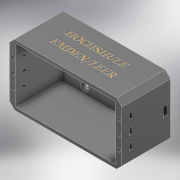
# Autodesk Inventor part: 3
Saved by Autodesk Inventor 2022 (Build 260153000, 153)
## iProperties
Company: HS Emden/Leer
Created: 2023-12-23
Part Number: 3
Material: PMMA-Kunststoff
Document SubType Name: Sheet Metal
Designer: Yaman Alsaady
Density: 1.188 g/cm^3
Appearance: Glatt - Schwarz
Sheet Metal Rule: Standard
Project: Delta-Robot
Author: Yaman Alsaady
Title: Case
## iProperties of the stored document 1_3D-Druck.ipt
Created: 2023-12-25
Part Number: 1_3D-Druck
Material: Generisch
Document SubType Name: Modeling
Designer: alsaa
Density: 1 g/cm^3
Appearance: Vorgabe
Author: alsaa
Autodesk Inventor part; units mm, degrees
(part 1 of 2)
ref_plane "YZ Plane" through (0, 0, 0) normal (1, 0, 0) x (0, 1, 0)
ref_plane "XZ Plane" through (0, 0, 0) normal (0, 1, 0) x (-1, 0, 0)
ref_plane "XY Plane" through (0, 0, 0) normal (0, 0, 1) x (1, 0, 0)
sketch "Skizze1" plane through (0, 0, 0) normal (0, 0, 1) x (1, 0, 0)
  line L0 (-30.75, -10.25) -> (10.25, -10.25)
  line L1 (10.25, -10.25) -> (10.25, 10.25)
  line L2 (10.25, 10.25) -> (-30.75, 10.25)
  line L3 (-30.75, 10.25) -> (-30.75, -10.25)
  line L4 (0, -10.25) -> (0, 10.25)
  circle A0 centre (-34.5, -5) radius 2.15
  circle A1 centre (-34.5, 5) radius 2.15
  circle A2 centre (14, 5) radius 2.15
  circle A3 centre (14, -5) radius 2.15
  line L5 (-10.25, -10.25) -> (-10.25, 10.25)
  line L6 (-56, 0) -> (56, 0)
  line L7 (53, 29) -> (-53, 29)
  line L8 (-53, 29) -> (-53, -29)
  line L9 (-53, -29) -> (53, -29)
  line L10 (53, -29) -> (53, 29)
  line L11 (53, 29) -> (-53, -29) construction
  line L12 (-53, 29) -> (53, -29) construction
  line L13 (-53, -10.25) -> (53, -10.25)
  line L14 (-53, 10.25) -> (53, 10.25)
  point P0 (0, 0)
  point P1 (0, 0)
  point P2 (0, 0)
  dimension "d8" = 48.5
  dimension "d9" = 4.3
  dimension "d10" = 20.5
  dimension "d11" = 41
  dimension "d12" = 34.5
  dimension "d13" = 10
  dimension "d14" = 58
  dimension "d15" = 106
  dimension "d18" = 20.5
  constraints: 30 end point, 6 midpoint, 6 parallel, 4 centre point, 4 horizontal, 4 point on line, 4 symmetric about line, 3 equal radius, 3 perpendicular, 2 coincident, 1 other
  measures "d8" distance of A2.centre A1.centre
  measures "d9" diameter of A0
  measures "d10" distance of L1.start L1.end
  measures "d11" distance of L0.start L1.start
  measures "d12" horizontal distance of L4.start A0.centre
  measures "d13" distance of A2.centre A3.centre
  measures "d14" distance of L9.end L7.start
  measures "d15" distance of L8.end L9.end
  measures "d18" distance between parallel lines of L14 L13
extrude "Extrusion1" add sketch "Skizze1" along normal blind 3 contours L3 L6 L5 L0 | L13 L8 L6 L3 | L0 L13 L10 L9 L8 | L5 L6 L4 L0 | L6 L8 L14 L3 | L3 L2 L5 L6 | L4 L6 L1 L0 | L5 L2 L4 L6 | L14 L8 L7 L10 L2 | L1 L6 L10 L13 | L4 L2 L1 L6 | L1 L14 L10 L6 | A0 | A1 | A2 | A3
sketch "Skizze2" plane through (0, 0, 3) normal (0, 0, 1) x (1, 0, 0)
  line L0 (53, 29) -> (-53, 29) projected
  line L1 (-53, -29) -> (53, -29) projected
  line L2 (-53, 29) -> (-47, 29)
  line L3 (-47, 29) -> (-47, -29)
  line L4 (-47, -29) -> (-53, -29)
  line L5 (-53, -29) -> (-53, 29)
  line L6 (53, -29) -> (53, 29) projected
  line L7 (53, 29) -> (47, 29)
  line L8 (47, 29) -> (47, -29)
  line L9 (47, -29) -> (53, -29)
  line L10 (53, -29) -> (53, 29)
  point P0 (0, 0)
  dimension "d19" = 6
  dimension "d20" = 6
  constraints: 16 end point, 4 parallel, 2 horizontal, 2 perpendicular, 2 point on line
  measures "d19" distance between parallel lines of L3 L5
  measures "d20" distance between parallel lines of L6 L8
extrude "Extrusion2" add sketch "Skizze2" along normal blind 43 contours L6 L1 L8 L0 | L3 L1 L5 L0
sketch "Skizze3" plane through (0, 0, 46) normal (0, 0, 1) x (1, 0, 0)
  line L0 (-47, 29) -> (-53, 29) construction
  line L1 (-53, 29) -> (-47, 29) construction
  line L2 (-47, 29) -> (-50, 29) construction
  line L3 (-50, 29) -> (-50, -29) construction
  line L4 (-53, 29) -> (-53, -29) construction
  line L5 (53, 29) -> (-53, 29) construction
  line L6 (0, 29) -> (0, -30.13) construction
  line L7 (-53, 0) -> (-47, 0) construction
  line L8 (-47, 29) -> (-47, -29) construction
  circle A0 centre (-50, 12.5) radius 1.85
  circle A1 centre (-50, -12.5) radius 1.85
  circle A2 centre (50, 12.5) radius 1.85
  circle A3 centre (50, -12.5) radius 1.85
  circle A4 centre (-50, 0) radius 1.85
  circle A5 centre (50, 0) radius 1.85
  point P0 (0, 0)
  dimension "d24" = 25
  dimension "d33" = 3.7
  constraints: 10 end point, 6 centre point, 5 midpoint, 4 symmetric about line, 2 equal length, 2 equal radius, 2 point on line, 1 vertical, 3 other
  measures "d24" distance of A1.centre A0.centre
  measures "d33" diameter of A4
extrude "Extrusion3" cut sketch "Skizze3" against normal blind 20
sketch "Skizze4" plane through (0, 0, 3) normal (0, 0, 1) x (1, 0, 0)
  line L0 (25, -20) -> (-25, -20)
  line L1 (-25, -20) -> (-25, 20)
  line L2 (-25, 20) -> (25, 20)
  line L3 (25, 20) -> (25, -20)
  line L4 (25, -20) -> (-25, 20) construction
  line L5 (-25, -20) -> (25, 20) construction
  circle A0 centre (-25, 20) radius 1.85
  circle A1 centre (25, 20) radius 1.85
  circle A2 centre (25, -20) radius 1.85
  circle A3 centre (-25, -20) radius 1.85
  point P0 (0, 0)
  dimension "d27" = 50
  dimension "d28" = 40
  dimension "d29" = 3.7
  constraints: 12 end point, 4 centre point, 4 coincident, 3 equal radius, 2 midpoint, 2 parallel, 1 horizontal, 1 perpendicular
  measures "d27" distance of L1.end L2.end
  measures "d28" distance of L2.end L0.start
  measures "d29" diameter of A1
extrude "Extrusion4" cut sketch "Skizze4" against normal through all contours A3 L1 L0 | L0 L1 A3 | A2 L3 L0 | L0 L3 A2 | A0 L2 L1 | L1 L2 A0 | A1 L2 L3 | L3 L2 A1
fillet "Rundung1" radius 2 4 edges at (-26.85, 20, 3) (23.15, 20, 3) (23.15, -20, 3) (-26.85, -20, 3)
sketch "Skizze5" plane through (0, 0, 3) normal (0, 0, 1) x (1, 0, 0)
  line L0 (-47, -29) -> (-47, 29) projected
  line L1 (-47, 26) -> (47, 26)
  line L2 (47, -29) -> (47, 29) projected
  line L3 (-47, -26) -> (47, -26)
  line L4 (-47, -29) -> (47, -29) projected
  line L5 (47, 29) -> (-47, 29) projected
  point P0 (0, 0)
  dimension "d34" = 3
  dimension "d35" = 3
  constraints: 4 end point, 2 horizontal, 2 point on line
  measures "d34" distance between parallel lines of L4 L3
  measures "d35" distance between parallel lines of L1 L5
extrude "Extrusion5" add sketch "Skizze5" along normal up to surface (43 mm away) contours L0 L3 L2 L4 | L0 L5 L2 L1
chamfer "Fase1" distance 5 angle 45 4 edges at (53, 29, 23) (53, -29, 23) (-53, -29, 23) (-53, 29, 23)
sketch "Skizze6" plane through (-48, -29, 0) normal (0, -1, 0) x (1, 0, 0)
  line L0 (0, 0) -> (0, 46) projected
  line L1 (0, 0) -> (96, 0) projected
  line L2 (96, 46) -> (96, 0) projected
  line L3 (0, 46) -> (96, 46) projected
  line L4 (0, 0) -> (0, 46) construction
  line L5 (0, 23) -> (96, 23) construction
  line L6 (1, 46) -> (95, 46) construction
  line L7 (48, 46) -> (48, 0) construction
  line L8 (75.5, 12) -> (20.5, 12) construction
  line L9 (20.5, 12) -> (20.5, 34) construction
  line L10 (20.5, 34) -> (75.5, 34) construction
  line L11 (75.5, 34) -> (75.5, 12) construction
  line L12 (77.3044, 18.1442) -> (76.7258, 17.963)
  spline S0 degree 2 poles (76.7258, 17.963) (76.6351, 17.9351) (76.4957, 17.8026) (76.4678, 17.712) knots 0 0 0 1 2 2 2
  line L13 (76.4678, 17.712) -> (75.4361, 13.0481)
  spline S1 degree 2 poles (75.4361, 13.0481) (75.4151, 12.9505) (75.4988, 12.8181) (75.5825, 12.7972) knots 0 0 0 1 2 2 2
  line L14 (75.5825, 12.7972) -> (76.1681, 12.6159)
  line L15 (76.1681, 12.6159) -> (76.1053, 12.3301)
  line L16 (76.1053, 12.3301) -> (73.2819, 12.3301)
  line L17 (73.2819, 12.3301) -> (73.3446, 12.6159)
  line L18 (73.3446, 12.6159) -> (73.9163, 12.7972)
  spline S2 degree 2 poles (73.9163, 12.7972) (74.0069, 12.825) (74.1533, 12.9505) (74.1742, 13.0481) knots 0 0 0 1 2 2 2
  line L19 (74.1742, 13.0481) -> (74.6065, 14.9932)
  line L20 (74.6065, 14.9932) -> (72.0828, 14.9932)
  line L21 (72.0828, 14.9932) -> (71.6506, 13.0481)
  spline S3 degree 2 poles (71.6506, 13.0481) (71.6297, 12.9505) (71.7133, 12.8181) (71.797, 12.7972) knots 0 0 0 1 2 2 2
  line L22 (71.797, 12.7972) -> (72.3826, 12.6159)
  line L23 (72.3826, 12.6159) -> (72.3198, 12.3301)
  line L24 (72.3198, 12.3301) -> (69.4964, 12.3301)
  line L25 (69.4964, 12.3301) -> (69.5591, 12.6159)
  line L26 (69.5591, 12.6159) -> (70.1308, 12.7972)
  spline S4 degree 2 poles (70.1308, 12.7972) (70.2214, 12.825) (70.3609, 12.9575) (70.3887, 13.0481) knots 0 0 0 1 2 2 2
  line L27 (70.3887, 13.0481) -> (71.4205, 17.712)
  spline S5 degree 2 poles (71.4205, 17.712) (71.4414, 17.8096) (71.3578, 17.9421) (71.2741, 17.963) knots 0 0 0 1 2 2 2
  line L28 (71.2741, 17.963) -> (70.6885, 18.1442)
  line L29 (70.6885, 18.1442) -> (70.7513, 18.4301)
  line L30 (70.7513, 18.4301) -> (73.5817, 18.4301)
  line L31 (73.5817, 18.4301) -> (73.5119, 18.1442)
  line L32 (73.5119, 18.1442) -> (72.9403, 17.963)
  spline S6 degree 2 poles (72.9403, 17.963) (72.8497, 17.9351) (72.7033, 17.8026) (72.6823, 17.712) knots 0 0 0 1 2 2 2
  line L33 (72.6823, 17.712) -> (72.2013, 15.523)
  line L34 (72.2013, 15.523) -> (74.718, 15.523)
  line L35 (74.718, 15.523) -> (75.206, 17.712)
  spline S7 degree 2 poles (75.206, 17.712) (75.2269, 17.8096) (75.1363, 17.9421) (75.0526, 17.963) knots 0 0 0 1 2 2 2
  line L36 (75.0526, 17.963) -> (74.474, 18.1442)
  line L37 (74.474, 18.1442) -> (74.5437, 18.4301)
  line L38 (74.5437, 18.4301) -> (77.3602, 18.4301)
  line L39 (77.3602, 18.4301) -> (77.3044, 18.1442)
  spline S8 degree 2 poles (67.1819, 18.5695) (67.7884, 18.5695) (68.7156, 18.2279) (69.343, 17.6005) (69.6777, 16.7081) (69.6777, 16.1504) knots 0 0 0 1 2 3 4 4 4
  spline S9 degree 2 poles (69.6777, 16.1504) (69.6777, 15.6694) (69.4685, 14.7143) (69.0572, 13.8359) (68.4437, 13.076) (67.6559, 12.5183) (66.6869, 12.1976) (66.1222, 12.1976) knots 0 0 0 1 2 3 4 5 6 6 6
  spline S10 degree 2 poles (66.1222, 12.1976) (65.4948, 12.1976) (64.5606, 12.5532) (63.9402, 13.1945) (63.6195, 14.0729) (63.6195, 14.6028) knots 0 0 0 1 2 3 4 4 4
  spline S11 degree 2 poles (63.6195, 14.6028) (63.6195, 15.042) (63.8077, 15.9692) (64.1981, 16.8476) (64.7977, 17.6353) (65.5854, 18.2209) (66.5823, 18.5695) (67.1819, 18.5695) knots 0 0 0 1 2 3 4 5 6 6 6
  spline S12 degree 2 poles (67.0494, 18.0606) (66.7148, 18.0606) (66.1362, 17.7469) (65.6761, 17.2101) (65.3275, 16.499) (65.1044, 15.6973) (64.9859, 14.8468) (64.9859, 14.4494) knots 0 0 0 1 2 3 4 5 6 6 6
  spline S13 degree 2 poles (64.9859, 14.4494) (64.9859, 14.045) (65.1323, 13.3967) (65.439, 12.9436) (65.9131, 12.6996) (66.2477, 12.6996) knots 0 0 0 1 2 3 4 4 4
  spline S14 degree 2 poles (66.2477, 12.6996) (66.5893, 12.6996) (67.1679, 13.0272) (67.6281, 13.578) (67.9697, 14.296) (68.1927, 15.0838) (68.3043, 15.8855) (68.3043, 16.248) knots 0 0 0 1 2 3 4 5 6 6 6
  spline S15 degree 2 poles (68.3043, 16.248) (68.3043, 16.6454) (68.1718, 17.3077) (67.8721, 17.7887) (67.398, 18.0606) (67.0494, 18.0606) knots 0 0 0 1 2 3 4 4 4
  spline S16 degree 2 poles (60.7682, 18.5556) (61.3468, 18.5556) (62.267, 18.1861) (62.9014, 17.5029) (63.2361, 16.5408) (63.2361, 15.9552) knots 0 0 0 1 2 3 4 4 4
  spline S17 degree 2 poles (63.2361, 15.9552) (63.2361, 15.4463) (62.999, 14.4842) (62.5668, 13.6477) (61.9394, 12.9645) (61.1655, 12.4695) (60.2453, 12.2046) (59.7294, 12.2046) knots 0 0 0 1 2 3 4 5 6 6 6
  spline S18 degree 2 poles (59.7294, 12.2046) (59.5063, 12.2046) (58.9695, 12.2673) (58.4537, 12.3649) (58.0005, 12.4974) (57.8402, 12.5601) knots 0 0 0 1 2 3 4 4 4
  line L40 (57.8402, 12.5601) -> (58.126, 14.0799)
  line L41 (58.126, 14.0799) -> (58.4676, 14.0799)
  line L42 (58.4676, 14.0799) -> (58.6419, 13.2852)
  spline S19 degree 2 poles (58.6419, 13.2852) (58.6489, 13.2154) (58.7186, 13.1248) (58.7743, 13.0969) knots 0 0 0 1 2 2 2
  spline S20 degree 2 poles (58.7743, 13.0969) (58.8929, 13.0342) (59.1996, 12.9017) (59.5273, 12.8041) (59.8549, 12.7484) (59.9943, 12.7484) knots 0 0 0 1 2 3 4 4 4
  spline S21 degree 2 poles (59.9943, 12.7484) (60.3708, 12.7484) (61.047, 13.2294) (61.5629, 14.059) (61.8627, 15.1744) (61.8627, 15.8158) knots 0 0 0 1 2 3 4 4 4
  spline S22 degree 2 poles (61.8627, 15.8158) (61.8627, 16.2759) (61.6954, 17.0288) (61.3119, 17.5656) (60.7054, 17.8445) (60.2662, 17.8445) knots 0 0 0 1 2 3 4 4 4
  spline S23 degree 2 poles (60.2662, 17.8445) (60.0222, 17.8445) (59.5203, 17.6911) (59.0532, 17.475) (58.6419, 17.2101) (58.4815, 17.0985) knots 0 0 0 1 2 3 4 4 4
  line L43 (58.4815, 17.0985) -> (58.2724, 17.0985)
  line L44 (58.2724, 17.0985) -> (58.3909, 17.6144)
  spline S24 degree 2 poles (58.3909, 17.6144) (58.5931, 17.7748) (59.0881, 18.1024) (59.6737, 18.3813) (60.3638, 18.5556) (60.7682, 18.5556) knots 0 0 0 1 2 3 4 4 4
  line L45 (58.2933, 18.1442) -> (57.7147, 17.963)
  spline S25 degree 2 poles (57.7147, 17.963) (57.6241, 17.9351) (57.4846, 17.8026) (57.4567, 17.712) knots 0 0 0 1 2 2 2
  line L46 (57.4567, 17.712) -> (56.425, 13.0481)
  spline S26 degree 2 poles (56.425, 13.0481) (56.4041, 12.9505) (56.4877, 12.8181) (56.5714, 12.7972) knots 0 0 0 1 2 2 2
  line L47 (56.5714, 12.7972) -> (57.157, 12.6159)
  line L48 (57.157, 12.6159) -> (57.0942, 12.3301)
  line L49 (57.0942, 12.3301) -> (54.2708, 12.3301)
  line L50 (54.2708, 12.3301) -> (54.3335, 12.6159)
  line L51 (54.3335, 12.6159) -> (54.9052, 12.7972)
  spline S27 degree 2 poles (54.9052, 12.7972) (54.9958, 12.825) (55.1422, 12.9505) (55.1631, 13.0481) knots 0 0 0 1 2 2 2
  line L52 (55.1631, 13.0481) -> (55.5954, 14.9932)
  line L53 (55.5954, 14.9932) -> (53.0717, 14.9932)
  line L54 (53.0717, 14.9932) -> (52.6395, 13.0481)
  spline S28 degree 2 poles (52.6395, 13.0481) (52.6186, 12.9505) (52.7022, 12.8181) (52.7859, 12.7972) knots 0 0 0 1 2 2 2
  line L55 (52.7859, 12.7972) -> (53.3715, 12.6159)
  line L56 (53.3715, 12.6159) -> (53.3087, 12.3301)
  line L57 (53.3087, 12.3301) -> (50.4853, 12.3301)
  line L58 (50.4853, 12.3301) -> (50.5481, 12.6159)
  line L59 (50.5481, 12.6159) -> (51.1197, 12.7972)
  spline S29 degree 2 poles (51.1197, 12.7972) (51.2103, 12.825) (51.3498, 12.9575) (51.3777, 13.0481) knots 0 0 0 1 2 2 2
  line L60 (51.3777, 13.0481) -> (52.4094, 17.712)
  spline S30 degree 2 poles (52.4094, 17.712) (52.4303, 17.8096) (52.3467, 17.9421) (52.263, 17.963) knots 0 0 0 1 2 2 2
  line L61 (52.263, 17.963) -> (51.6774, 18.1442)
  line L62 (51.6774, 18.1442) -> (51.7402, 18.4301)
  line L63 (51.7402, 18.4301) -> (54.5706, 18.4301)
  line L64 (54.5706, 18.4301) -> (54.5009, 18.1442)
  line L65 (54.5009, 18.1442) -> (53.9292, 17.963)
  spline S31 degree 2 poles (53.9292, 17.963) (53.8386, 17.9351) (53.6922, 17.8026) (53.6713, 17.712) knots 0 0 0 1 2 2 2
  line L66 (53.6713, 17.712) -> (53.1902, 15.523)
  line L67 (53.1902, 15.523) -> (55.7069, 15.523)
  line L68 (55.7069, 15.523) -> (56.1949, 17.712)
  spline S32 degree 2 poles (56.1949, 17.712) (56.2158, 17.8096) (56.1252, 17.9421) (56.0415, 17.963) knots 0 0 0 1 2 2 2
  line L69 (56.0415, 17.963) -> (55.4629, 18.1442)
  line L70 (55.4629, 18.1442) -> (55.5326, 18.4301)
  line L71 (55.5326, 18.4301) -> (58.3491, 18.4301)
  line L72 (58.3491, 18.4301) -> (58.2933, 18.1442)
  spline S33 degree 2 poles (48.9028, 18.5695) (49.1607, 18.5695) (49.7045, 18.5068) (50.2622, 18.3952) (50.799, 18.2488) (51.0361, 18.1652) knots 0 0 0 1 2 3 4 4 4
  line L73 (51.0361, 18.1652) -> (50.7433, 16.4362)
  line L74 (50.7433, 16.4362) -> (50.3947, 16.4362)
  line L75 (50.3947, 16.4362) -> (50.2204, 17.3077)
  spline S34 degree 2 poles (50.2204, 17.3077) (50.2065, 17.3704) (50.1367, 17.482) (50.074, 17.5308) knots 0 0 0 1 2 2 2
  spline S35 degree 2 poles (50.074, 17.5308) (49.9415, 17.6353) (49.5233, 17.8166) (49.098, 17.9421) (48.7076, 18.0118) (48.5961, 18.0118) knots 0 0 0 1 2 3 4 4 4
  spline S36 degree 2 poles (48.5961, 18.0118) (48.359, 18.0118) (47.9129, 17.8724) (47.5573, 17.6005) (47.3412, 17.2101) (47.3412, 16.9452) knots 0 0 0 1 2 3 4 4 4
  spline S37 degree 2 poles (47.3412, 16.9452) (47.3412, 16.7639) (47.4667, 16.492) (47.6758, 16.2829) (47.9547, 16.1156) (48.1011, 16.0458) knots 0 0 0 1 2 3 4 4 4
  spline S38 degree 2 poles (48.1011, 16.0458) (48.3521, 15.9204) (48.8679, 15.6833) (49.1259, 15.5648) knots 0 0 0 1 2 2 2
  spline S39 degree 2 poles (49.1259, 15.5648) (49.3559, 15.4602) (49.7254, 15.1814) (49.9903, 14.8328) (50.1298, 14.3936) (50.1298, 14.1287) knots 0 0 0 1 2 3 4 4 4
  spline S40 degree 2 poles (50.1298, 14.1287) (50.1298, 13.808) (49.9206, 13.2712) (49.5581, 12.846) (49.0771, 12.5253) (48.5263, 12.3022) (47.9477, 12.1976) (47.6619, 12.1976) knots 0 0 0 1 2 3 4 5 6 6 6
  spline S41 degree 2 poles (47.6619, 12.1976) (47.4039, 12.1976) (46.902, 12.2464) (46.4001, 12.337) (45.9051, 12.4625) (45.6611, 12.5322) knots 0 0 0 1 2 3 4 4 4
  line L76 (45.6611, 12.5322) -> (45.9887, 14.1287)
  line L77 (45.9887, 14.1287) -> (46.3303, 14.1287)
  line L78 (46.3303, 14.1287) -> (46.4837, 13.313)
  spline S42 degree 2 poles (46.4837, 13.313) (46.5116, 13.2015) (46.6301, 13.1039) knots 0 0 0 1 1 1
  spline S43 degree 2 poles (46.6301, 13.1039) (46.7486, 13.0202) (47.0763, 12.8808) (47.4179, 12.7972) (47.7246, 12.7484) (47.8153, 12.7484) knots 0 0 0 1 2 3 4 4 4
  spline S44 degree 2 poles (47.8153, 12.7484) (48.0314, 12.7484) (48.4218, 12.9017) (48.7076, 13.1876) (48.8679, 13.564) (48.8679, 13.7871) knots 0 0 0 1 2 3 4 4 4
  spline S45 degree 2 poles (48.8679, 13.7871) (48.8679, 13.9684) (48.7355, 14.2402) (48.5124, 14.4424) (48.2266, 14.6028) (48.0662, 14.6794) knots 0 0 0 1 2 3 4 4 4
  spline S46 degree 2 poles (48.0662, 14.6794) (47.8222, 14.798) (47.3133, 15.021) (47.0693, 15.1465) knots 0 0 0 1 2 2 2
  spline S47 degree 2 poles (47.0693, 15.1465) (46.8393, 15.265) (46.4628, 15.5369) (46.1979, 15.8785) (46.0585, 16.3108) (46.0585, 16.5826) knots 0 0 0 1 2 3 4 4 4
  spline S48 degree 2 poles (46.0585, 16.5826) (46.0585, 16.9521) (46.3094, 17.5308) (46.7347, 17.97) (47.2994, 18.2767) (47.9338, 18.4789) (48.5891, 18.5695) (48.9028, 18.5695) knots 0 0 0 1 2 3 4 5 6 6 6
  line L79 (45.926, 18.1442) -> (45.3474, 17.963)
  spline S49 degree 2 poles (45.3474, 17.963) (45.2567, 17.9351) (45.1173, 17.8026) (45.0894, 17.712) knots 0 0 0 1 2 2 2
  line L80 (45.0894, 17.712) -> (44.0577, 13.0481)
  spline S50 degree 2 poles (44.0577, 13.0481) (44.0367, 12.9505) (44.1204, 12.8181) (44.2041, 12.7972) knots 0 0 0 1 2 2 2
  line L81 (44.2041, 12.7972) -> (44.7897, 12.6159)
  line L82 (44.7897, 12.6159) -> (44.7269, 12.3301)
  line L83 (44.7269, 12.3301) -> (41.9035, 12.3301)
  line L84 (41.9035, 12.3301) -> (41.9662, 12.6159)
  line L85 (41.9662, 12.6159) -> (42.5379, 12.7972)
  spline S51 degree 2 poles (42.5379, 12.7972) (42.6285, 12.825) (42.7749, 12.9505) (42.7958, 13.0481) knots 0 0 0 1 2 2 2
  line L86 (42.7958, 13.0481) -> (43.2281, 14.9932)
  line L87 (43.2281, 14.9932) -> (40.7044, 14.9932)
  line L88 (40.7044, 14.9932) -> (40.2722, 13.0481)
  spline S52 degree 2 poles (40.2722, 13.0481) (40.2513, 12.9505) (40.3349, 12.8181) (40.4186, 12.7972) knots 0 0 0 1 2 2 2
  line L89 (40.4186, 12.7972) -> (41.0042, 12.6159)
  line L90 (41.0042, 12.6159) -> (40.9414, 12.3301)
  line L91 (40.9414, 12.3301) -> (38.118, 12.3301)
  line L92 (38.118, 12.3301) -> (38.1807, 12.6159)
  line L93 (38.1807, 12.6159) -> (38.7524, 12.7972)
  spline S53 degree 2 poles (38.7524, 12.7972) (38.843, 12.825) (38.9825, 12.9575) (39.0103, 13.0481) knots 0 0 0 1 2 2 2
  line L94 (39.0103, 13.0481) -> (40.0421, 17.712)
  spline S54 degree 2 poles (40.0421, 17.712) (40.063, 17.8096) (39.9794, 17.9421) (39.8957, 17.963) knots 0 0 0 1 2 2 2
  line L95 (39.8957, 17.963) -> (39.3101, 18.1442)
  line L96 (39.3101, 18.1442) -> (39.3729, 18.4301)
  line L97 (39.3729, 18.4301) -> (42.2033, 18.4301)
  line L98 (42.2033, 18.4301) -> (42.1335, 18.1442)
  line L99 (42.1335, 18.1442) -> (41.5619, 17.963)
  spline S55 degree 2 poles (41.5619, 17.963) (41.4713, 17.9351) (41.3249, 17.8026) (41.3039, 17.712) knots 0 0 0 1 2 2 2
  line L100 (41.3039, 17.712) -> (40.8229, 15.523)
  line L101 (40.8229, 15.523) -> (43.3396, 15.523)
  line L102 (43.3396, 15.523) -> (43.8276, 17.712)
  spline S56 degree 2 poles (43.8276, 17.712) (43.8485, 17.8096) (43.7579, 17.9421) (43.6742, 17.963) knots 0 0 0 1 2 2 2
  line L103 (43.6742, 17.963) -> (43.0956, 18.1442)
  line L104 (43.0956, 18.1442) -> (43.1653, 18.4301)
  line L105 (43.1653, 18.4301) -> (45.9818, 18.4301)
  line L106 (45.9818, 18.4301) -> (45.926, 18.1442)
  spline S57 degree 2 poles (35.8593, 18.5695) (36.3751, 18.5695) (37.149, 18.3116) (37.6718, 17.8933) (37.9298, 17.3286) (37.9298, 17.0218) knots 0 0 0 1 2 3 4 4 4
  spline S58 degree 2 poles (37.9298, 17.0218) (37.9298, 16.973) (37.9158, 16.8266) (37.8949, 16.6593) (37.874, 16.506) (37.8601, 16.4502) knots 0 0 0 1 2 3 4 4 4
  line L107 (37.8601, 16.4502) -> (37.1002, 13.0481)
  spline S59 degree 2 poles (37.1002, 13.0481) (37.0793, 12.9505) (37.1629, 12.8181) (37.2466, 12.7972) knots 0 0 0 1 2 2 2
  line L108 (37.2466, 12.7972) -> (37.8322, 12.6159)
  line L109 (37.8322, 12.6159) -> (37.7694, 12.3301)
  line L110 (37.7694, 12.3301) -> (34.946, 12.3301)
  line L111 (34.946, 12.3301) -> (35.0087, 12.6159)
  line L112 (35.0087, 12.6159) -> (35.5804, 12.7972)
  spline S60 degree 2 poles (35.5804, 12.7972) (35.671, 12.825) (35.8174, 12.9436) (35.8383, 13.0481) knots 0 0 0 1 2 2 2
  line L113 (35.8383, 13.0481) -> (36.5634, 16.3526)
  spline S61 degree 2 poles (36.5634, 16.3526) (36.5773, 16.4153) (36.5982, 16.5687) (36.6122, 16.7151) (36.6261, 16.8615) (36.6261, 16.9033) knots 0 0 0 1 2 3 4 4 4
  spline S62 degree 2 poles (36.6261, 16.9033) (36.6261, 17.0916) (36.5285, 17.4471) (36.2706, 17.7399) (35.8244, 17.9212) (35.4758, 17.9212) knots 0 0 0 1 2 3 4 4 4
  spline S63 degree 2 poles (35.4758, 17.9212) (35.0436, 17.9212) (34.4441, 17.6214) (34.0397, 17.1613) (33.8166, 16.6175) (33.7609, 16.3665) knots 0 0 0 1 2 3 4 4 4
  line L114 (33.7609, 16.3665) -> (33.0289, 13.076)
  spline S64 degree 2 poles (33.0289, 13.076) (33.0079, 12.9784) (33.0846, 12.8599) (33.1753, 12.825) knots 0 0 0 1 2 2 2
  line L115 (33.1753, 12.825) -> (33.7539, 12.6159)
  line L116 (33.7539, 12.6159) -> (33.6911, 12.3301)
  line L117 (33.6911, 12.3301) -> (31.4951, 12.3301)
  line L118 (31.4951, 12.3301) -> (31.5579, 12.6159)
  line L119 (31.5579, 12.6159) -> (32.1365, 12.825)
  spline S65 degree 2 poles (32.1365, 12.825) (32.2271, 12.8599) (32.3735, 12.9784) (32.3945, 13.076) knots 0 0 0 1 2 2 2
  line L120 (32.3945, 13.076) -> (33.1404, 16.4362)
  spline S66 degree 2 poles (33.1404, 16.4362) (33.238, 16.8545) (33.5796, 17.4959) (34.0258, 17.97) (34.5347, 18.2906) (35.0785, 18.4858) (35.6153, 18.5695) (35.8593, 18.5695) knots 0 0 0 1 2 3 4 5 6 6 6
  line L121 (32.3945, 18.1442) -> (31.8158, 17.963)
  spline S67 degree 2 poles (31.8158, 17.963) (31.7182, 17.9351) (31.5858, 17.8026) (31.5649, 17.712) knots 0 0 0 1 2 2 2
  line L122 (31.5649, 17.712) -> (30.5331, 13.0481)
  spline S68 degree 2 poles (30.5331, 13.0481) (30.5122, 12.9505) (30.5889, 12.8181) (30.6725, 12.7972) knots 0 0 0 1 2 2 2
  line L123 (30.6725, 12.7972) -> (31.2581, 12.6159)
  line L124 (31.2581, 12.6159) -> (31.1954, 12.3301)
  line L125 (31.1954, 12.3301) -> (28.3301, 12.3301)
  line L126 (28.3301, 12.3301) -> (28.3929, 12.6159)
  line L127 (28.3929, 12.6159) -> (28.9924, 12.7972)
  spline S69 degree 2 poles (28.9924, 12.7972) (29.083, 12.825) (29.2225, 12.9575) (29.2503, 13.0481) knots 0 0 0 1 2 2 2
  line L128 (29.2503, 13.0481) -> (30.3239, 17.9002)
  line L129 (30.3239, 17.9002) -> (28.2534, 17.9002)
  spline S70 degree 2 poles (28.2534, 17.9002) (28.2186, 17.9002) (28.1419, 17.8514) (28.0791, 17.7887) (28.0303, 17.712) (28.0164, 17.6772) knots 0 0 0 1 2 3 4 4 4
  line L130 (28.0164, 17.6772) -> (27.3959, 16.492)
  line L131 (27.3959, 16.492) -> (27.0474, 16.492)
  line L132 (27.0474, 16.492) -> (27.4796, 18.4301)
  line L133 (27.4796, 18.4301) -> (32.4572, 18.4301)
  line L134 (32.4572, 18.4301) -> (32.3945, 18.1442)
  line L135 (27.1798, 18.1442) -> (26.5942, 17.963)
  spline S71 degree 2 poles (26.5942, 17.963) (26.5036, 17.9351) (26.3642, 17.8026) (26.3363, 17.712) knots 0 0 0 1 2 2 2
  line L136 (26.3363, 17.712) -> (25.3045, 13.0481)
  spline S72 degree 2 poles (25.3045, 13.0481) (25.2836, 12.9505) (25.3673, 12.8181) (25.4509, 12.7972) knots 0 0 0 1 2 2 2
  line L137 (25.4509, 12.7972) -> (26.0435, 12.6159)
  line L138 (26.0435, 12.6159) -> (25.9807, 12.3301)
  line L139 (25.9807, 12.3301) -> (21.0519, 12.3301)
  line L140 (21.0519, 12.3301) -> (21.4075, 13.9335)
  line L141 (21.4075, 13.9335) -> (21.763, 13.9335)
  line L142 (21.763, 13.9335) -> (21.8955, 13.0133)
  spline S73 degree 2 poles (21.8955, 13.0133) (21.9025, 12.9436) (21.9652, 12.8599) (22.0419, 12.8599) knots 0 0 0 1 2 2 2
  line L143 (22.0419, 12.8599) -> (23.9939, 12.8599)
  line L144 (23.9939, 12.8599) -> (24.4749, 14.9932)
  line L145 (24.4749, 14.9932) -> (23.2479, 14.9932)
  spline S74 degree 2 poles (23.2479, 14.9932) (23.1573, 14.9932) (23.0597, 14.9165) (23.0179, 14.8468) knots 0 0 0 1 2 2 2
  line L146 (23.0179, 14.8468) -> (22.5717, 14.1287)
  line L147 (22.5717, 14.1287) -> (22.265, 14.1287)
  line L148 (22.265, 14.1287) -> (22.7599, 16.3805)
  line L149 (22.7599, 16.3805) -> (23.0737, 16.3805)
  line L150 (23.0737, 16.3805) -> (23.1991, 15.6694)
  spline S75 degree 2 poles (23.1991, 15.6694) (23.2131, 15.5997) (23.2689, 15.509) (23.3525, 15.509) knots 0 0 0 1 2 2 2
  line L151 (23.3525, 15.509) -> (24.5865, 15.509)
  line L152 (24.5865, 15.509) -> (25.1163, 17.9002)
  line L153 (25.1163, 17.9002) -> (22.7042, 17.9002)
  spline S76 degree 2 poles (22.7042, 17.9002) (22.6205, 17.9002) (22.5229, 17.8166) (22.4881, 17.7469) knots 0 0 0 1 2 2 2
  line L154 (22.4881, 17.7469) -> (21.9303, 16.7012)
  line L155 (21.9303, 16.7012) -> (21.5748, 16.7012)
  line L156 (21.5748, 16.7012) -> (21.9582, 18.4301)
  line L157 (21.9582, 18.4301) -> (27.2426, 18.4301)
  line L158 (27.2426, 18.4301) -> (27.1798, 18.1442)
  line L159 (78.1445, 31.6831) -> (77.5589, 31.5018)
  spline S77 degree 2 poles (77.5589, 31.5018) (77.4682, 31.4739) (77.3288, 31.3415) (77.3009, 31.2508) knots 0 0 0 1 2 2 2
  line L160 (77.3009, 31.2508) -> (76.2691, 26.587)
  spline S78 degree 2 poles (76.2691, 26.587) (76.2482, 26.4894) (76.3319, 26.3569) (76.4155, 26.336) knots 0 0 0 1 2 2 2
  line L161 (76.4155, 26.336) -> (77.0081, 26.1547)
  line L162 (77.0081, 26.1547) -> (76.9454, 25.8689)
  line L163 (76.9454, 25.8689) -> (72.0166, 25.8689)
  line L164 (72.0166, 25.8689) -> (72.3721, 27.4723)
  line L165 (72.3721, 27.4723) -> (72.7277, 27.4723)
  line L166 (72.7277, 27.4723) -> (72.8601, 26.5521)
  spline S79 degree 2 poles (72.8601, 26.5521) (72.8671, 26.4824) (72.9298, 26.3987) (73.0065, 26.3987) knots 0 0 0 1 2 2 2
  line L167 (73.0065, 26.3987) -> (74.9585, 26.3987)
  line L168 (74.9585, 26.3987) -> (75.4395, 28.532)
  line L169 (75.4395, 28.532) -> (74.2126, 28.532)
  spline S80 degree 2 poles (74.2126, 28.532) (74.1219, 28.532) (74.0243, 28.4553) (73.9825, 28.3856) knots 0 0 0 1 2 2 2
  line L170 (73.9825, 28.3856) -> (73.5363, 27.6675)
  line L171 (73.5363, 27.6675) -> (73.2296, 27.6675)
  line L172 (73.2296, 27.6675) -> (73.7246, 29.9193)
  line L173 (73.7246, 29.9193) -> (74.0383, 29.9193)
  line L174 (74.0383, 29.9193) -> (74.1638, 29.2082)
  spline S81 degree 2 poles (74.1638, 29.2082) (74.1777, 29.1385) (74.2335, 29.0479) (74.3171, 29.0479) knots 0 0 0 1 2 2 2
  line L175 (74.3171, 29.0479) -> (75.5511, 29.0479)
  line L176 (75.5511, 29.0479) -> (76.0809, 31.4391)
  line L177 (76.0809, 31.4391) -> (73.6688, 31.4391)
  spline S82 degree 2 poles (73.6688, 31.4391) (73.5851, 31.4391) (73.4875, 31.3554) (73.4527, 31.2857) knots 0 0 0 1 2 2 2
  line L178 (73.4527, 31.2857) -> (72.895, 30.24)
  line L179 (72.895, 30.24) -> (72.5394, 30.24)
  line L180 (72.5394, 30.24) -> (72.9229, 31.9689)
  line L181 (72.9229, 31.9689) -> (78.2072, 31.9689)
  line L182 (78.2072, 31.9689) -> (78.1445, 31.6831)
  line L183 (72.4488, 31.6831) -> (71.8702, 31.4739)
  spline S83 degree 2 poles (71.8702, 31.4739) (71.7726, 31.4391) (71.6331, 31.3136) (71.6122, 31.223) knots 0 0 0 1 2 2 2
  line L184 (71.6122, 31.223) -> (70.5874, 26.587)
  spline S84 degree 2 poles (70.5874, 26.587) (70.5665, 26.4894) (70.6571, 26.3569) (70.7269, 26.336) knots 0 0 0 1 2 2 2
  line L185 (70.7269, 26.336) -> (71.3125, 26.1547)
  line L186 (71.3125, 26.1547) -> (71.2497, 25.8689)
  line L187 (71.2497, 25.8689) -> (68.9491, 25.8689)
  line L188 (68.9491, 25.8689) -> (68.4333, 29.3337)
  line L189 (68.4333, 29.3337) -> (68.3287, 30.2051)
  line L190 (68.3287, 30.2051) -> (68.3147, 30.2051)
  line L191 (68.3147, 30.2051) -> (65.7702, 25.8689)
  line L192 (65.7702, 25.8689) -> (63.5045, 25.8689)
  line L193 (63.5045, 25.8689) -> (63.5672, 26.1547)
  line L194 (63.5672, 26.1547) -> (64.1389, 26.336)
  spline S85 degree 2 poles (64.1389, 26.336) (64.2295, 26.3639) (64.3759, 26.4963) (64.3968, 26.587) knots 0 0 0 1 2 2 2
  line L195 (64.3968, 26.587) -> (65.4286, 31.2508)
  spline S86 degree 2 poles (65.4286, 31.2508) (65.4565, 31.3484) (65.3728, 31.4739) (65.2891, 31.5018) knots 0 0 0 1 2 2 2
  line L196 (65.2891, 31.5018) -> (64.7035, 31.6831)
  line L197 (64.7035, 31.6831) -> (64.7663, 31.9689)
  line L198 (64.7663, 31.9689) -> (67.5897, 31.9689)
  line L199 (67.5897, 31.9689) -> (67.527, 31.6831)
  line L200 (67.527, 31.6831) -> (66.9553, 31.5018)
  spline S87 degree 2 poles (66.9553, 31.5018) (66.8577, 31.4739) (66.7183, 31.3415) (66.6974, 31.2508) knots 0 0 0 1 2 2 2
  line L201 (66.6974, 31.2508) -> (65.7074, 26.7891)
  line L202 (65.7074, 26.7891) -> (65.7214, 26.7891)
  line L203 (65.7214, 26.7891) -> (66.1536, 27.5769)
  line L204 (66.1536, 27.5769) -> (68.1614, 30.965)
  line L205 (68.1614, 30.965) -> (68.8167, 31.9689)
  line L206 (68.8167, 31.9689) -> (69.2768, 31.9689)
  line L207 (69.2768, 31.9689) -> (69.9251, 27.5769)
  line L208 (69.9251, 27.5769) -> (70.0158, 26.7752)
  line L209 (70.0158, 26.7752) -> (70.0297, 26.7752)
  line L210 (70.0297, 26.7752) -> (71.0127, 31.223)
  spline S88 degree 2 poles (71.0127, 31.223) (71.0406, 31.3206) (70.9569, 31.446) (70.8733, 31.4739) knots 0 0 0 1 2 2 2
  line L211 (70.8733, 31.4739) -> (70.2877, 31.6831)
  line L212 (70.2877, 31.6831) -> (70.3504, 31.9689)
  line L213 (70.3504, 31.9689) -> (72.5115, 31.9689)
  line L214 (72.5115, 31.9689) -> (72.4488, 31.6831)
  line L215 (64.2434, 31.6831) -> (63.6578, 31.5018)
  spline S89 degree 2 poles (63.6578, 31.5018) (63.5602, 31.4739) (63.4278, 31.3415) (63.3999, 31.2508) knots 0 0 0 1 2 2 2
  line L216 (63.3999, 31.2508) -> (62.3681, 26.587)
  spline S90 degree 2 poles (62.3681, 26.587) (62.3472, 26.4894) (62.4239, 26.3569) (62.5145, 26.336) knots 0 0 0 1 2 2 2
  line L217 (62.5145, 26.336) -> (63.1001, 26.1547)
  line L218 (63.1001, 26.1547) -> (63.0374, 25.8689)
  line L219 (63.0374, 25.8689) -> (60.2837, 25.8689)
  spline S91 degree 2 poles (60.2837, 25.8689) (60.0118, 25.8689) (59.4053, 25.9665) (58.8127, 26.1826) (58.2759, 26.5451) (57.8715, 27.0819) (57.6275, 27.807) (57.6275, 28.274) knots 0 0 0 1 2 3 4 5 6 6 6
  spline S92 degree 2 poles (57.6275, 28.274) (57.6275, 28.9015) (57.9134, 29.9263) (58.4153, 30.7489) (59.1125, 31.3624) (59.9351, 31.7667) (60.8483, 31.9689) (61.3224, 31.9689) knots 0 0 0 1 2 3 4 5 6 6 6
  line L220 (61.3224, 31.9689) -> (64.2992, 31.9689)
  line L221 (64.2992, 31.9689) -> (64.2434, 31.6831)
  spline S93 degree 2 poles (61.2736, 31.453) (60.939, 31.453) (60.3325, 31.2369) (59.8235, 30.8535) (59.4331, 30.2958) (59.1473, 29.6265) (59.0079, 28.8387) (59.0079, 28.4065) knots 0 0 0 1 2 3 4 5 6 6 6
  spline S94 degree 2 poles (59.0079, 28.4065) (59.0079, 27.9464) (59.217, 27.2004) (59.6283, 26.6706) (60.2279, 26.3848) (60.6113, 26.3848) knots 0 0 0 1 2 3 4 4 4
  line L222 (60.6113, 26.3848) -> (61.0575, 26.3848)
  line L223 (61.0575, 26.3848) -> (62.1799, 31.453)
  line L224 (62.1799, 31.453) -> (61.2736, 31.453)
  line L225 (57.8088, 31.6831) -> (57.2232, 31.5018)
  spline S95 degree 2 poles (57.2232, 31.5018) (57.1326, 31.4739) (56.9931, 31.3415) (56.9653, 31.2508) knots 0 0 0 1 2 2 2
  line L226 (56.9653, 31.2508) -> (55.9335, 26.587)
  spline S96 degree 2 poles (55.9335, 26.587) (55.9126, 26.4894) (55.9962, 26.3569) (56.0799, 26.336) knots 0 0 0 1 2 2 2
  line L227 (56.0799, 26.336) -> (56.6725, 26.1547)
  line L228 (56.6725, 26.1547) -> (56.6097, 25.8689)
  line L229 (56.6097, 25.8689) -> (51.6809, 25.8689)
  line L230 (51.6809, 25.8689) -> (52.0365, 27.4723)
  line L231 (52.0365, 27.4723) -> (52.392, 27.4723)
  line L232 (52.392, 27.4723) -> (52.5245, 26.5521)
  spline S97 degree 2 poles (52.5245, 26.5521) (52.5314, 26.4824) (52.5942, 26.3987) (52.6709, 26.3987) knots 0 0 0 1 2 2 2
  line L233 (52.6709, 26.3987) -> (54.6229, 26.3987)
  line L234 (54.6229, 26.3987) -> (55.1039, 28.532)
  line L235 (55.1039, 28.532) -> (53.8769, 28.532)
  spline S98 degree 2 poles (53.8769, 28.532) (53.7863, 28.532) (53.6887, 28.4553) (53.6469, 28.3856) knots 0 0 0 1 2 2 2
  line L236 (53.6469, 28.3856) -> (53.2007, 27.6675)
  line L237 (53.2007, 27.6675) -> (52.8939, 27.6675)
  line L238 (52.8939, 27.6675) -> (53.3889, 29.9193)
  line L239 (53.3889, 29.9193) -> (53.7026, 29.9193)
  line L240 (53.7026, 29.9193) -> (53.8281, 29.2082)
  spline S99 degree 2 poles (53.8281, 29.2082) (53.8421, 29.1385) (53.8978, 29.0479) (53.9815, 29.0479) knots 0 0 0 1 2 2 2
  line L241 (53.9815, 29.0479) -> (55.2154, 29.0479)
  line L242 (55.2154, 29.0479) -> (55.7453, 31.4391)
  line L243 (55.7453, 31.4391) -> (53.3331, 31.4391)
  spline S100 degree 2 poles (53.3331, 31.4391) (53.2495, 31.4391) (53.1519, 31.3554) (53.117, 31.2857) knots 0 0 0 1 2 2 2
  line L244 (53.117, 31.2857) -> (52.5593, 30.24)
  line L245 (52.5593, 30.24) -> (52.2038, 30.24)
  line L246 (52.2038, 30.24) -> (52.5872, 31.9689)
  line L247 (52.5872, 31.9689) -> (57.8715, 31.9689)
  line L248 (57.8715, 31.9689) -> (57.8088, 31.6831)
  line L249 (49.4361, 27.8558) -> (49.7359, 27.2004)
  line L250 (49.7359, 27.2004) -> (49.7498, 27.2004)
  line L251 (49.7498, 27.2004) -> (50.6422, 31.223)
  spline S101 degree 2 poles (50.6422, 31.223) (50.6701, 31.3206) (50.5864, 31.4391) (50.5027, 31.4739) knots 0 0 0 1 2 2 2
  line L252 (50.5027, 31.4739) -> (49.9171, 31.6831)
  line L253 (49.9171, 31.6831) -> (49.9799, 31.9689)
  line L254 (49.9799, 31.9689) -> (52.1759, 31.9689)
  line L255 (52.1759, 31.9689) -> (52.1131, 31.6831)
  line L256 (52.1131, 31.6831) -> (51.5345, 31.4739)
  spline S102 degree 2 poles (51.5345, 31.4739) (51.4369, 31.4391) (51.2975, 31.3136) (51.2766, 31.223) knots 0 0 0 1 2 2 2
  line L257 (51.2766, 31.223) -> (50.2587, 26.6009)
  spline S103 degree 2 poles (50.2587, 26.6009) (50.2378, 26.5033) (50.3215, 26.3708) (50.4051, 26.3499) knots 0 0 0 1 2 2 2
  line L258 (50.4051, 26.3499) -> (51.0256, 26.1547)
  line L259 (51.0256, 26.1547) -> (50.9559, 25.8689)
  line L260 (50.9559, 25.8689) -> (49.0248, 25.8689)
  line L261 (49.0248, 25.8689) -> (47.2262, 29.6823)
  line L262 (47.2262, 29.6823) -> (46.9613, 30.2748)
  line L263 (46.9613, 30.2748) -> (46.9473, 30.2748)
  line L264 (46.9473, 30.2748) -> (46.1386, 26.6079)
  spline S104 degree 2 poles (46.1386, 26.6079) (46.1177, 26.5172) (46.1874, 26.3918) (46.285, 26.3639) knots 0 0 0 1 2 2 2
  line L265 (46.285, 26.3639) -> (46.8846, 26.1547)
  line L266 (46.8846, 26.1547) -> (46.8218, 25.8689)
  line L267 (46.8218, 25.8689) -> (44.6189, 25.8689)
  line L268 (44.6189, 25.8689) -> (44.6816, 26.1547)
  line L269 (44.6816, 26.1547) -> (45.2393, 26.3639)
  spline S105 degree 2 poles (45.2393, 26.3639) (45.3369, 26.3987) (45.4763, 26.5172) (45.4973, 26.6079) knots 0 0 0 1 2 2 2
  line L270 (45.4973, 26.6079) -> (46.4663, 30.965)
  line L271 (46.4663, 30.965) -> (46.8288, 32.0107)
  line L272 (46.8288, 32.0107) -> (47.4702, 32.0107)
  line L273 (47.4702, 32.0107) -> (49.4361, 27.8558)
  line L274 (41.3283, 25.3809) -> (40.5615, 25.3809)
  line L275 (40.5615, 25.3809) -> (45.4345, 33.8024)
  line L276 (45.4345, 33.8024) -> (46.1735, 33.8024)
  line L277 (46.1735, 33.8024) -> (41.3283, 25.3809)
  line L278 (41.2586, 31.6831) -> (40.68, 31.5018)
  spline S106 degree 2 poles (40.68, 31.5018) (40.5824, 31.4739) (40.4499, 31.3415) (40.429, 31.2508) knots 0 0 0 1 2 2 2
  line L279 (40.429, 31.2508) -> (39.3973, 26.587)
  spline S107 degree 2 poles (39.3973, 26.587) (39.3763, 26.4894) (39.453, 26.3569) (39.5367, 26.336) knots 0 0 0 1 2 2 2
  line L280 (39.5367, 26.336) -> (40.1223, 26.1547)
  line L281 (40.1223, 26.1547) -> (40.0595, 25.8689)
  line L282 (40.0595, 25.8689) -> (37.1943, 25.8689)
  line L283 (37.1943, 25.8689) -> (37.257, 26.1547)
  line L284 (37.257, 26.1547) -> (37.8566, 26.336)
  spline S108 degree 2 poles (37.8566, 26.336) (37.9472, 26.3639) (38.0866, 26.4963) (38.1145, 26.587) knots 0 0 0 1 2 2 2
  line L285 (38.1145, 26.587) -> (39.1881, 31.4391)
  line L286 (39.1881, 31.4391) -> (37.1176, 31.4391)
  spline S109 degree 2 poles (37.1176, 31.4391) (37.0827, 31.4391) (37.0061, 31.3903) (36.9433, 31.3275) (36.8945, 31.2508) (36.8806, 31.216) knots 0 0 0 1 2 3 4 4 4
  line L287 (36.8806, 31.216) -> (36.2601, 30.0308)
  line L288 (36.2601, 30.0308) -> (35.9115, 30.0308)
  line L289 (35.9115, 30.0308) -> (36.3438, 31.9689)
  line L290 (36.3438, 31.9689) -> (41.3214, 31.9689)
  line L291 (41.3214, 31.9689) -> (41.2586, 31.6831)
  line L292 (36.044, 31.6831) -> (35.4584, 31.5018)
  spline S110 degree 2 poles (35.4584, 31.5018) (35.3678, 31.4739) (35.2283, 31.3415) (35.2005, 31.2508) knots 0 0 0 1 2 2 2
  line L293 (35.2005, 31.2508) -> (34.1687, 26.587)
  spline S111 degree 2 poles (34.1687, 26.587) (34.1478, 26.4894) (34.2314, 26.3569) (34.3151, 26.336) knots 0 0 0 1 2 2 2
  line L294 (34.3151, 26.336) -> (34.9077, 26.1547)
  line L295 (34.9077, 26.1547) -> (34.8449, 25.8689)
  line L296 (34.8449, 25.8689) -> (29.9161, 25.8689)
  line L297 (29.9161, 25.8689) -> (30.2717, 27.4723)
  line L298 (30.2717, 27.4723) -> (30.6272, 27.4723)
  line L299 (30.6272, 27.4723) -> (30.7597, 26.5521)
  spline S112 degree 2 poles (30.7597, 26.5521) (30.7666, 26.4824) (30.8294, 26.3987) (30.9061, 26.3987) knots 0 0 0 1 2 2 2
  line L300 (30.9061, 26.3987) -> (32.8581, 26.3987)
  line L301 (32.8581, 26.3987) -> (33.3391, 28.532)
  line L302 (33.3391, 28.532) -> (32.1121, 28.532)
  spline S113 degree 2 poles (32.1121, 28.532) (32.0215, 28.532) (31.9239, 28.4553) (31.8821, 28.3856) knots 0 0 0 1 2 2 2
  line L303 (31.8821, 28.3856) -> (31.4359, 27.6675)
  line L304 (31.4359, 27.6675) -> (31.1291, 27.6675)
  line L305 (31.1291, 27.6675) -> (31.6241, 29.9193)
  line L306 (31.6241, 29.9193) -> (31.9378, 29.9193)
  line L307 (31.9378, 29.9193) -> (32.0633, 29.2082)
  spline S114 degree 2 poles (32.0633, 29.2082) (32.0773, 29.1385) (32.133, 29.0479) (32.2167, 29.0479) knots 0 0 0 1 2 2 2
  line L308 (32.2167, 29.0479) -> (33.4506, 29.0479)
  line L309 (33.4506, 29.0479) -> (33.9805, 31.4391)
  line L310 (33.9805, 31.4391) -> (31.5683, 31.4391)
  spline S115 degree 2 poles (31.5683, 31.4391) (31.4847, 31.4391) (31.3871, 31.3554) (31.3522, 31.2857) knots 0 0 0 1 2 2 2
  line L311 (31.3522, 31.2857) -> (30.7945, 30.24)
  line L312 (30.7945, 30.24) -> (30.439, 30.24)
  line L313 (30.439, 30.24) -> (30.8224, 31.9689)
  line L314 (30.8224, 31.9689) -> (36.1067, 31.9689)
  line L315 (36.1067, 31.9689) -> (36.044, 31.6831)
  line L316 (30.3623, 31.6831) -> (29.7767, 31.5018)
  spline S116 degree 2 poles (29.7767, 31.5018) (29.6861, 31.4739) (29.5466, 31.3415) (29.5187, 31.2508) knots 0 0 0 1 2 2 2
  line L317 (29.5187, 31.2508) -> (28.487, 26.587)
  spline S117 degree 2 poles (28.487, 26.587) (28.4661, 26.4894) (28.5497, 26.3569) (28.6334, 26.336) knots 0 0 0 1 2 2 2
  line L318 (28.6334, 26.336) -> (29.2259, 26.1547)
  line L319 (29.2259, 26.1547) -> (29.1632, 25.8689)
  line L320 (29.1632, 25.8689) -> (24.2344, 25.8689)
  line L321 (24.2344, 25.8689) -> (24.5899, 27.4723)
  line L322 (24.5899, 27.4723) -> (24.9455, 27.4723)
  line L323 (24.9455, 27.4723) -> (25.0779, 26.5521)
  spline S118 degree 2 poles (25.0779, 26.5521) (25.0849, 26.4824) (25.1477, 26.3987) (25.2243, 26.3987) knots 0 0 0 1 2 2 2
  line L324 (25.2243, 26.3987) -> (27.1763, 26.3987)
  line L325 (27.1763, 26.3987) -> (27.6574, 28.532)
  line L326 (27.6574, 28.532) -> (26.4304, 28.532)
  spline S119 degree 2 poles (26.4304, 28.532) (26.3398, 28.532) (26.2422, 28.4553) (26.2003, 28.3856) knots 0 0 0 1 2 2 2
  line L327 (26.2003, 28.3856) -> (25.7542, 27.6675)
  line L328 (25.7542, 27.6675) -> (25.4474, 27.6675)
  line L329 (25.4474, 27.6675) -> (25.9424, 29.9193)
  line L330 (25.9424, 29.9193) -> (26.2561, 29.9193)
  line L331 (26.2561, 29.9193) -> (26.3816, 29.2082)
  spline S120 degree 2 poles (26.3816, 29.2082) (26.3955, 29.1385) (26.4513, 29.0479) (26.535, 29.0479) knots 0 0 0 1 2 2 2
  line L332 (26.535, 29.0479) -> (27.7689, 29.0479)
  line L333 (27.7689, 29.0479) -> (28.2987, 31.4391)
  line L334 (28.2987, 31.4391) -> (25.8866, 31.4391)
  spline S121 degree 2 poles (25.8866, 31.4391) (25.803, 31.4391) (25.7054, 31.3554) (25.6705, 31.2857) knots 0 0 0 1 2 2 2
  line L335 (25.6705, 31.2857) -> (25.1128, 30.24)
  line L336 (25.1128, 30.24) -> (24.7573, 30.24)
  line L337 (24.7573, 30.24) -> (25.1407, 31.9689)
  line L338 (25.1407, 31.9689) -> (30.425, 31.9689)
  line L339 (30.425, 31.9689) -> (30.3623, 31.6831)
  line L340 (24.6736, 31.6831) -> (24.095, 31.5018)
  spline S122 degree 2 poles (24.095, 31.5018) (24.0113, 31.4739) (23.8649, 31.3415) (23.837, 31.2508) knots 0 0 0 1 2 2 2
  line L341 (23.837, 31.2508) -> (22.8053, 26.587)
  spline S123 degree 2 poles (22.8053, 26.587) (22.7843, 26.4894) (22.868, 26.3569) (22.9517, 26.336) knots 0 0 0 1 2 2 2
  line L342 (22.9517, 26.336) -> (23.5373, 26.1547)
  line L343 (23.5373, 26.1547) -> (23.4815, 25.8689)
  line L344 (23.4815, 25.8689) -> (20.6999, 25.8689)
  spline S124 degree 2 poles (20.6999, 25.8689) (20.0934, 25.8689) (19.3195, 26.1129) (18.8734, 26.5172) (18.6991, 27.0122) (18.6991, 27.2632) knots 0 0 0 1 2 3 4 4 4
  spline S125 degree 2 poles (18.6991, 27.2632) (18.6991, 27.5351) (18.8455, 27.9952) (19.0965, 28.3716) (19.4381, 28.6644) (19.8215, 28.8875) (20.2328, 29.0339) (20.435, 29.0688) knots 0 0 0 1 2 3 4 5 6 6 6
  line L345 (20.435, 29.0688) -> (19.2847, 31.202)
  spline S126 degree 2 poles (19.2847, 31.202) (19.2359, 31.2996) (19.0477, 31.4739) (18.964, 31.5018) knots 0 0 0 1 2 2 2
  line L346 (18.964, 31.5018) -> (18.3645, 31.6831)
  line L347 (18.3645, 31.6831) -> (18.4272, 31.9689)
  line L348 (18.4272, 31.9689) -> (19.7727, 31.9689)
  spline S127 degree 2 poles (19.7727, 31.9689) (19.9679, 31.9689) (20.2049, 31.9131) (20.3792, 31.7876) (20.5047, 31.5715) (20.5814, 31.4182) knots 0 0 0 1 2 3 4 4 4
  line L349 (20.5814, 31.4182) -> (21.6131, 29.3895)
  line L350 (21.6131, 29.3895) -> (22.136, 29.2431)
  line L351 (22.136, 29.2431) -> (22.5752, 31.2508)
  spline S128 degree 2 poles (22.5752, 31.2508) (22.5961, 31.3484) (22.5055, 31.4809) (22.4218, 31.5018) knots 0 0 0 1 2 2 2
  line L352 (22.4218, 31.5018) -> (21.8153, 31.6831)
  line L353 (21.8153, 31.6831) -> (21.885, 31.9689)
  line L354 (21.885, 31.9689) -> (24.7294, 31.9689)
  line L355 (24.7294, 31.9689) -> (24.6736, 31.6831)
  spline S129 degree 2 poles (21.5295, 28.8387) (21.167, 28.8387) (20.6162, 28.6017) (20.2607, 28.1974) (20.0864, 27.6606) (20.0864, 27.3678) knots 0 0 0 1 2 3 4 4 4
  spline S130 degree 2 poles (20.0864, 27.3678) (20.0864, 27.1168) (20.2258, 26.7473) (20.5117, 26.5033) (20.9369, 26.3848) (21.2227, 26.3848) knots 0 0 0 1 2 3 4 4 4
  line L356 (21.2227, 26.3848) -> (21.4946, 26.3848)
  line L357 (21.4946, 26.3848) -> (22.0314, 28.7969)
  spline S131 degree 2 poles (22.0314, 28.7969) (21.9966, 28.8039) (21.8571, 28.8178) (21.6968, 28.8318) (21.5643, 28.8387) (21.5295, 28.8387) knots 0 0 0 1 2 3 4 4 4
  point P0 (48, 23)
  point P1 (75.5, 23)
  point P2 (48, 12)
  point P3 (20.5, 23)
  dimension "d41" = 22
  dimension "d42" = 55
  constraints: 7 midpoint, 4 end point, 3 point on line, 1 vertical, 2 other
  measures "d41" distance of L8.end L9.end
  measures "d42" distance of L8.start L8.end
extrude "Extrusion6" cut sketch "Skizze6" against normal blind 0.5 contours L12 S0 L13 S1 L14 L15 L16 L17 L18 S2 L19 L20 L21 S3 L22 L23 L24 L25 L26 S4 L27 S5 L28 L29 L30 L31 L32 S6 L33 L34 L35 S7 L36 L37 L38 L39 | S8 S9 S10 S11 | S16 S17 S18 L40 L41 L42 S19 S20 S21 S22 S23 L43 L44 S24 | L45 S25 L46 S26 L47 L48 L49 L50 L51 S27 L52 L53 L54 S28 L55 L56 L57 L58 L59 S29 L60 S30 L61 L62 L63 L64 L65 S31 L66 L67 L68 S32 L69 L70 L71 L72 | S33 L73 L74 L75 S34 S35 S36 S37 S38 S39 S40 S41 L76 L77 L78 S42 S43 S44 S45 S46 S47 S48 | L79 S49 L80 S50 L81 L82 L83 L84 L85 S51 L86 L87 L88 S52 L89 L90 L91 L92 L93 S53 L94 S54 L95 L96 L97 L98 L99 S55 L100 L101 L102 S56 L103 L104 L105 L106 | S57 S58 L107 S59 L108 L109 L110 L111 L112 S60 L113 S61 S62 S63 L114 S64 L115 L116 L117 L118 L119 S65 L120 S66 | L121 S67 L122 S68 L123 L124 L125 L126 L127 S69 L128 L129 S70 L130 L131 L132 L133 L134 | L135 S71 L136 S72 L137 L138 L139 L140 L141 L142 S73 L143 L144 L145 S74 L146 L147 L148 L149 L150 S75 L151 L152 L153 S76 L154 L155 L156 L157 L158 | L159 S77 L160 S78 L161 L162 L163 L164 L165 L166 S79 L167 L168 L169 S80 L170 L171 L172 L173 L174 S81 L175 L176 L177 S82 L178 L179 L180 L181 L182 | L183 S83 L184 S84 L185 L186 L187 L188 L189 L190 L191 L192 L193 L194 S85 L195 S86 L196 L197 L198 L199 L200 S87 L201 L202 L203 L204 L205 L206 L207 L208 L209 L210 S88 L211 L212 L213 L214 | L215 S89 L216 S90 L217 L218 L219 S91 S92 L220 L221 | L225 S95 L226 S96 L227 L228 L229 L230 L231 L232 S97 L233 L234 L235 S98 L236 L237 L238 L239 L240 S99 L241 L242 L243 S100 L244 L245 L246 L247 L248 | L249 L250 L251 S101 L252 L253 L254 L255 L256 S102 L257 S103 L258 L259 L260 L261 L262 L263 L264 S104 L265 L266 L267 L268 L269 S105 L270 L271 L272 L273 | L274 L275 L276 L277 | L278 S106 L279 S107 L280 L281 L282 L283 L284 S108 L285 L286 S109 L287 L288 L289 L290 L291 | L292 S110 L293 S111 L294 L295 L296 L297 L298 L299 S112 L300 L301 L302 S113 L303 L304 L305 L306 L307 S114 L308 L309 L310 S115 L311 L312 L313 L314 L315 | L316 S116 L317 S117 L318 L319 L320 L321 L322 L323 S118 L324 L325 L326 S119 L327 L328 L329 L330 L331 S120 L332 L333 L334 S121 L335 L336 L337 L338 L339 | L340 S122 L341 S123 L342 L343 L344 S124 S125 L345 S126 L346 L347 L348 S127 L349 L350 L351 S128 L352 L353 L354 L355
pattern_circular "Runde Anordnung1" count 2 over 360 about axis through (0, 0, -10) along (0, 0, 1) of "Extrusion6"